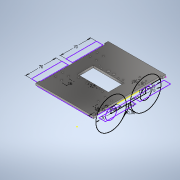
# Autodesk Inventor part: maze_02
Saved by Autodesk Inventor 2020 (Build 240168000, 168)
## iProperties
Created: 2022-07-14
Part Number: maze_02
Material: Сталь нержавеющая, 440C
Document SubType Name: Modeling
Designer: akapu
Density: 7.75 g/cm^3
Appearance: Сталь — полированная
Author: akapu
Autodesk Inventor part; units mm, degrees
ref_plane "YZ Plane" through (0, 0, 0) normal (1, 0, 0) x (0, 1, 0)
ref_plane "XZ Plane" through (0, 0, 0) normal (0, 1, 0) x (-1, 0, 0)
ref_plane "XY Plane" through (0, 0, 0) normal (0, 0, 1) x (1, 0, 0)
sketch "Эскиз2" plane through (0, 0, 0) normal (0, 1, 0) x (-1, 0, 0)
  line L0 (-37, -102) -> (-37, -192)
  line L1 (-166, -192) -> (-163, -192)
  line L2 (-163, -192) -> (-163, -102)
  line L3 (-37, -192) -> (-34, -192)
  line L4 (-34, -200) -> (-166, -200)
  line L5 (-37, -98) -> (-37, -102)
  line L6 (-163, -98) -> (-163, -102)
  line L7 (-166, -192) -> (-166, -200)
  line L8 (-34, -192) -> (-34, -200)
  line L9 (-163, -192) -> (-163, -157)
  line L10 (-163, -157) -> (-37, -157)
  line L11 (-163, -157) -> (-163, -63)
  line L12 (-163, -63) -> (-37, -63)
  line L13 (-34, -34.5) -> (-166, -34.5)
  line L14 (-166, -34.5) -> (-163, -34.5)
  line L15 (-163, -42.5) -> (-166, -42.5)
  line L16 (-166, -42.5) -> (-166, -34.5)
  line L17 (-34, -34.5) -> (-37, -34.5)
  line L18 (-37, -42.5) -> (-34, -42.5)
  line L19 (-37, -98) -> (-37, -34.5)
  line L20 (-34, -34.5) -> (-34, -42.5)
  line L21 (-163, -63) -> (-163, -34.5)
  point P0 (-37, -63)
  dimension "d181" = 94
  dimension "d247" = 8
  constraints: 44 end point, 5 parallel, 4 point on line, 3 horizontal, 3 perpendicular, 3 vertical
  measures "d181" distance of L9.end L11.end
  measures "d247" distance of L14.end L15.start
extrude "Выдавливание1" add sketch "Эскиз2" along normal blind 5
sketch "Эскиз3" plane through (0, 5, 0) normal (0, 1, 0) x (1, 0, 0)
  line L0 (163, 42.5) -> (163, 34.5)
  line L1 (34, 34.5) -> (166, 34.5) projected
  line L2 (156, 77.5) -> (156, 69.5)
  line L3 (166, 200) -> (34, 200) projected
  line L4 (156, 157) -> (156, 149)
  line L5 (156, 149) -> (142, 149)
  line L6 (142, 149) -> (142, 165)
  line L7 (142, 165) -> (156, 165)
  line L8 (156, 165) -> (156, 149)
  line L9 (156, 69.5) -> (142, 69.5)
  line L10 (142, 69.5) -> (142, 85.5)
  line L11 (142, 85.5) -> (156, 85.5)
  line L12 (156, 85.5) -> (156, 69.5)
  line L13 (37, 192) -> (37, 42.5) projected
  line L14 (44, 165) -> (58, 165)
  line L15 (58, 165) -> (58, 149)
  line L16 (58, 149) -> (44, 149)
  line L17 (44, 149) -> (44, 165)
  line L18 (58, 85.5) -> (44, 85.5)
  line L19 (44, 85.5) -> (44, 69.5)
  line L20 (44, 69.5) -> (58, 69.5)
  line L21 (58, 69.5) -> (58, 85.5)
  circle A0 centre (156, 69.5) radius 1.6
  circle A1 centre (142, 69.5) radius 1.6
  circle A2 centre (142, 85.5) radius 1.6
  circle A3 centre (156, 85.5) radius 1.6
  circle A4 centre (58, 69.5) radius 1.6
  circle A5 centre (58, 85.5) radius 1.6
  circle A6 centre (44, 69.5) radius 1.6
  circle A7 centre (44, 85.5) radius 1.6
  circle A8 centre (58, 149) radius 1.6
  circle A9 centre (58, 165) radius 1.6
  circle A10 centre (44, 149) radius 1.6
  circle A11 centre (44, 165) radius 1.6
  circle A12 centre (142, 165) radius 1.6
  circle A13 centre (142, 149) radius 1.6
  circle A14 centre (156, 149) radius 1.6
  circle A15 centre (156, 165) radius 1.6
  point P0 (0, 0)
  point P1 (37, 63)
  dimension "d255" = 14
  dimension "d256" = 16
  dimension "d260" = 14
  dimension "d261" = 3.2
  dimension "d262" = 3.2
  dimension "d263" = 3.2
  dimension "d264" = 3.2
  dimension "d265" = 3.2
  dimension "d266" = 3.2
  dimension "d267" = 3.2
  dimension "d268" = 3.2
  dimension "d269" = 3.2
  dimension "d270" = 3.2
  dimension "d271" = 3.2
  dimension "d272" = 3.2
  dimension "d273" = 3.2
  dimension "d274" = 3.2
  dimension "d275" = 3.2
  dimension "d276" = 3.2
  constraints: 38 end point, 16 centre point, 16 coincident, 8 parallel, 4 horizontal, 4 perpendicular, 3 point on line, 1 vertical
  measures "d255" distance of L6.end L7.end
  measures "d256" distance of L5.end L6.end
  measures "d260" distance of L15.end L16.end
  measures "d261" diameter of A0
  measures "d262" diameter of A1
  measures "d263" diameter of A2
  measures "d264" diameter of A3
  measures "d265" diameter of A4
  measures "d266" diameter of A5
  measures "d267" diameter of A6
  measures "d268" diameter of A7
  measures "d269" diameter of A8
  measures "d270" diameter of A9
  measures "d271" diameter of A10
  measures "d272" diameter of A11
  measures "d273" diameter of A12
  measures "d274" diameter of A13
  measures "d275" diameter of A14
  measures "d276" diameter of A15
extrude "Выдавливание2" cut sketch "Эскиз3" against normal blind 5 contours A0 L9 L2 | L2 L9 A0 | A3 L11 L12 | L12 L11 A3 | A1 L10 L9 | L9 L10 A1 | A2 L10 L11 | L11 L10 A2 | A14 L5 L4 | L4 L5 A14 | A15 L7 L8 | L8 L7 A15 | A13 L6 L5 | L5 L6 A13 | A12 L6 L7 | L7 L6 A12 | L17 A11 L14 | L14 A11 L17 | A9 L15 L14 | L14 L15 A9 | A10 L16 L17 | L17 L16 A10 | A8 L16 L15 | L15 L16 A8 | A7 L19 L18 | L18 L19 A7 | A5 L21 L18 | L18 L21 A5 | A6 L20 L19 | L19 L20 A6 | A4 L20 L21 | L21 L20 A4
sketch "Эскиз4" plane through (0, 0, 0) normal (0, -1, 0) x (1, 0, 0)
  line L0 (166, -200) -> (34, -200) projected
  line L1 (163, -157) -> (163, -170)
  line L2 (163, -170) -> (101.2, -170)
  line L3 (101.2, -170) -> (101.2, -144)
  line L4 (101.2, -144) -> (163, -144)
  line L5 (163, -144) -> (163, -170)
  line L6 (37, -170) -> (98.8, -170)
  line L7 (98.8, -170) -> (98.8, -144)
  line L8 (98.8, -144) -> (37, -144)
  line L9 (37, -144) -> (37, -170)
  line L10 (156, -157) -> (156, -165)
  line L11 (156, -165) -> (142, -165)
  line L12 (142, -165) -> (142, -149)
  line L13 (142, -149) -> (156, -149)
  line L14 (156, -149) -> (156, -165)
  line L15 (44, -165) -> (58, -165)
  line L16 (58, -165) -> (58, -149)
  line L17 (58, -149) -> (44, -149)
  line L18 (44, -149) -> (44, -165)
  line L19 (101.2, -144) -> (106.2, -144)
  line L20 (106.2, -90.5) -> (101.2, -90.5)
  line L21 (163, -41) -> (163, -192) projected
  line L22 (101.2, -90.5) -> (163, -90.5)
  line L23 (163, -90.5) -> (163, -64.5)
  line L24 (163, -64.5) -> (101.2, -64.5)
  line L25 (101.2, -64.5) -> (101.2, -90.5)
  line L26 (37, -192) -> (37, -42.5) projected
  line L27 (98.8, -90.5) -> (37, -90.5)
  line L28 (37, -90.5) -> (37, -64.5)
  line L29 (37, -64.5) -> (98.8, -64.5)
  line L30 (98.8, -64.5) -> (98.8, -90.5)
  line L31 (44, -77.5) -> (44, -85.5)
  circle A0 centre (58, -71) radius 1.6 projected
  line L32 (44, -85.5) -> (58.5568, -85.5)
  line L33 (58.5568, -85.5) -> (58.5568, -69.5)
  line L34 (58.5568, -69.5) -> (44, -69.5)
  line L35 (44, -69.5) -> (44, -85.5)
  circle A1 centre (142, -71) radius 1.6 projected
  line L36 (156, -85.5) -> (142, -85.5)
  line L37 (142, -85.5) -> (142, -69.4)
  line L38 (142, -69.4) -> (156, -69.4)
  line L39 (156, -69.4) -> (156, -85.5)
  line L40 (163, -77.5) -> (163, -34.5)
  line L41 (163, -34.5) -> (37, -34.5)
  line L42 (37, -34.5) -> (37, -41)
  line L43 (163, -157) -> (170, -157)
  line L44 (170, -157) -> (170, -192)
  line L45 (163, -77.5) -> (170, -77.5)
  line L46 (170, -77.5) -> (170, -42.5)
  line L47 (37, -77.5) -> (30, -77.5)
  line L48 (30, -77.5) -> (30, -42.5)
  line L49 (30, -42.5) -> (15, -42.5)
  line L50 (15, -42.5) -> (15, -112.5)
  line L51 (15, -112.5) -> (30, -112.5)
  line L52 (30, -112.5) -> (30, -42.5)
  line L53 (170, -42.5) -> (185, -42.5)
  line L54 (185, -42.5) -> (185, -112.5)
  line L55 (185, -112.5) -> (170, -112.5)
  line L56 (170, -112.5) -> (170, -42.5)
  line L57 (37, -157) -> (30, -157)
  line L58 (30, -192) -> (15, -192)
  line L59 (15, -192) -> (15, -122)
  line L60 (15, -122) -> (30, -122)
  line L61 (30, -122) -> (30, -192)
  line L62 (170, -192) -> (185, -192)
  line L63 (185, -192) -> (185, -122)
  line L64 (185, -122) -> (170, -122)
  line L65 (170, -122) -> (170, -192)
  point P0 (142, -155)
  point P1 (44, -155)
  point P2 (37, -63)
  dimension "d162" = 8
  dimension "d163" = 16
  dimension "d240" = 26
  dimension "d241" = 2.4
  dimension "d243" = 16
  dimension "d244" = 14
  dimension "d245" = 43
  dimension "d284" = 70
  dimension "d286" = 70
  constraints: 126 end point, 25 parallel, 17 perpendicular, 14 horizontal, 7 point on line, 2 midpoint, 1 vertical, 1 vertical alignment, 3 other
  measures "d162" distance of L10.start L10.end
  measures "d163" distance of L11.end L12.end
  measures "d240" distance of L23.end L22.end
  measures "d241" distance of L20.end L27.start
  measures "d243" distance of L33.end L32.end
  measures "d244" distance of L37.end L38.end
  measures "d245" distance of L40.start L40.end
  measures "d284" distance of L50.end L49.end
  measures "d286" distance of L58.end L59.end
sketch "Эскиз11" plane through (163, 0, -42.5) normal (1, 0, 0) x (0, 0, -1)
  line L0 (0, 0) -> (149.5, 0) projected
  line L1 (0, 0) -> (35, 0)
  line L2 (35, 0) -> (35, -12.5)
  line L3 (149.5, 0) -> (114.5, 0)
  line L4 (114.5, 0) -> (114.5, -12.5)
  line L5 (114.5, -12.5) -> (35, -12.5)
  circle A0 centre (35, -12.5) radius 35
  circle A1 centre (114.5, -12.5) radius 35
  line L6 (59.7487, -37.2487) -> (74.75, -22.2475)
  line L7 (74.75, -22.2475) -> (89.7513, -37.2487)
  line L8 (74.75, -22.2475) -> (74.75, -12.5)
  circle A2 centre (35, -12.5) radius 12.5
  circle A3 centre (114.5, -12.5) radius 12.5
  point P0 (-42.5, 0)
  dimension "d291" = 70
  dimension "d292" = 70
  dimension "d287" = 35
  dimension "d288" = 12.5
  dimension "d289" = 35
  dimension "d290" = 12.5
  dimension "d321" = 90
  dimension "d322" = 9.7475
  constraints: 16 end point, 3 coincident, 2 perpendicular, 2 point on line, 2 vertical alignment, 1 midpoint, 12 other
  measures "d287" distance of L0.start L1.end
  measures "d288" distance of L1.end L2.end
  measures "d289" distance of L0.end L3.end
  measures "d290" distance of L3.end L4.end
  measures "d321" angle of L7 L6
  measures "d322" distance of L6.end L8.end
sketch "Эскиз12" plane through (0, 0, 0) normal (0, -1, 0) x (1, 0, 0)
  line L0 (37, -192) -> (37, -42.5) projected
  line L1 (34, -34.5) -> (166, -34.5) projected
  line L2 (37, -34.5) -> (37, -77.5)
  line L3 (37, -77.5) -> (98.8, -77.5)
  line L4 (98.8, -77.5) -> (98.8, -90.5)
  line L5 (98.8, -90.5) -> (93.8, -90.5)
  line L6 (100, -99.25) -> (64.5, -99.25)
  line L7 (64.5, -99.25) -> (135.5, -99.25)
  line L8 (135.5, -99.25) -> (135.5, -135.25)
  line L9 (135.5, -135.25) -> (64.5, -135.25)
  line L10 (64.5, -135.25) -> (64.5, -99.25)
  line L11 (106.2, -141) -> (93.8, -141)
  circle A0 centre (106.2, -141) radius 3
  circle A1 centre (93.8, -141) radius 3
  line L12 (106.2, -93.5) -> (93.8, -93.5)
  circle A2 centre (106.2, -93.5) radius 3
  circle A3 centre (93.8, -93.5) radius 3
  point P0 (0, 0)
  dimension "d296" = 43
  dimension "d298" = 13
  dimension "d310" = 35.5
  dimension "d311" = 71
  dimension "d312" = 36
  dimension "d343" = 6
  dimension "d344" = 6
  dimension "d346" = 6
  dimension "d347" = 6
  constraints: 22 end point, 4 centre point, 4 coincident, 4 perpendicular, 2 parallel, 2 point on line, 1 horizontal
  measures "d296" distance of L2.start L2.end
  measures "d298" distance of L3.end L4.end
  measures "d310" distance of L6.start L6.end
  measures "d311" distance of L8.end L9.end
  measures "d312" distance of L7.end L8.end
  measures "d343" diameter of A0
  measures "d344" diameter of A1
  measures "d346" diameter of A2
  measures "d347" diameter of A3
extrude "Выдавливание9" cut sketch "Эскиз12" against normal blind 5
sketch "Эскиз13" plane through (0, 0, 0) normal (0, -1, 0) x (1, 0, 0)
  line L0 (135.5, -135.25) -> (135.5, -99.25) projected
  line L1 (135.5, -99.25) -> (135.5, -90.5)
  line L2 (135.5, -135.25) -> (64.5, -135.25) projected
  line L3 (64.5, -135.25) -> (64.5, -144)
  line L4 (64.5, -144) -> (135.5, -144)
  line L5 (135.5, -144) -> (135.5, -90.5)
  line L6 (135.5, -90.5) -> (64.5, -90.5)
  line L7 (64.5, -90.5) -> (64.5, -144)
  line L8 (135.5, -90.5) -> (127.5, -90.5)
  line L9 (127.5, -90.5) -> (127.5, -93.5)
  line L10 (127.5, -93.5) -> (135.5, -93.5)
  line L11 (135.5, -93.5) -> (135.5, -90.5)
  line L12 (64.5, -144) -> (72.5, -144)
  line L13 (72.5, -144) -> (72.5, -141)
  line L14 (72.5, -141) -> (64.5, -141)
  line L15 (64.5, -141) -> (64.5, -144)
  line L16 (72.5, -141) -> (127.5, -141)
  line L17 (127.5, -141) -> (127.5, -93.5)
  line L18 (127.5, -93.5) -> (72.5, -93.5)
  line L19 (72.5, -93.5) -> (72.5, -141)
  circle A0 centre (127.5, -93.5) radius 1.6
  circle A1 centre (127.5, -141) radius 1.6
  circle A2 centre (72.5, -141) radius 1.6
  circle A3 centre (72.5, -93.5) radius 1.6
  point P0 (163, -42.5)
  dimension "d325" = 8.75
  dimension "d326" = 8.75
  dimension "d327" = 8
  dimension "d328" = 3
  dimension "d329" = 8
  dimension "d330" = 3
  dimension "d331" = 3.2
  dimension "d332" = 3.2
  dimension "d333" = 3.2
  dimension "d334" = 3.2
  constraints: 36 end point, 8 parallel, 4 centre point, 4 coincident, 4 horizontal, 4 perpendicular, 2 vertical
  measures "d325" distance of L0.end L1.end
  measures "d326" distance of L2.end L3.end
  measures "d327" distance of L10.end L9.end
  measures "d328" distance of L9.end L8.end
  measures "d329" distance of L14.end L13.end
  measures "d330" distance of L13.end L12.end
  measures "d331" diameter of A0
  measures "d332" diameter of A1
  measures "d333" diameter of A2
  measures "d334" diameter of A3
extrude "Выдавливание10" cut sketch "Эскиз13" against normal blind 5 contours A1 L16 L17 | L17 L16 A1 | A0 L18 L17 | L17 L10 A0 | L10 L9 A0 | A3 L18 L19 | L19 L18 A3 | A2 L16 L19 | L19 L14 A2 | L18 A0 L9 | A2 L14 L13 | L13 L16 A2
sketch "Эскиз15" plane through (0, 5, 0) normal (0, 1, 0) x (1, 0, 0)
  line L0 (72.5, 93.5) -> (80.5, 93.5)
  line L1 (80.5, 93.5) -> (80.5, 96.3)
  line L2 (80.5, 96.3) -> (72.5, 96.3)
  line L3 (72.5, 96.3) -> (72.5, 93.5)
  circle A0 centre (127.5, 93.5) radius 1.6 projected
  line L4 (127.5, 93.5) -> (119.5, 93.5)
  line L5 (119.5, 93.5) -> (119.5, 96.3)
  line L6 (119.5, 96.3) -> (127.5, 96.3)
  line L7 (127.5, 96.3) -> (127.5, 93.5)
  circle A1 centre (127.5, 141) radius 1.6 projected
  line L8 (127.5, 141) -> (119.5, 141)
  line L9 (119.5, 141) -> (119.5, 138.2)
  line L10 (119.5, 138.2) -> (127.5, 138.2)
  line L11 (127.5, 138.2) -> (127.5, 141)
  line L12 (72.5, 141) -> (80.5, 141)
  line L13 (80.5, 141) -> (80.5, 138.2)
  line L14 (80.5, 138.2) -> (72.5, 138.2)
  line L15 (72.5, 138.2) -> (72.5, 141)
  circle A2 centre (80.5, 138.2) radius 1.6
  circle A3 centre (119.5, 138.2) radius 1.6
  circle A4 centre (119.5, 96.3) radius 1.6
  circle A5 centre (80.5, 96.3) radius 1.6
  point P0 (0, 0)
  dimension "d348" = 8
  dimension "d349" = 2.8
  dimension "d350" = 8
  dimension "d351" = 2.8
  dimension "d352" = 8
  dimension "d353" = 2.8
  dimension "d354" = 3.2
  dimension "d355" = 3.2
  dimension "d356" = 3.2
  dimension "d357" = 3.2
  constraints: 32 end point, 8 parallel, 4 centre point, 4 coincident, 4 horizontal, 4 perpendicular, 4 point on line
  measures "d348" distance of L2.end L1.end
  measures "d349" distance of L1.end L0.end
  measures "d350" distance of L5.end L6.end
  measures "d351" distance of L4.end L5.end
  measures "d352" distance of L10.end L9.end
  measures "d353" distance of L9.end L8.end
  measures "d354" diameter of A2
  measures "d355" diameter of A3
  measures "d356" diameter of A4
  measures "d357" diameter of A5
extrude "Выдавливание12" cut sketch "Эскиз15" against normal blind 5 contours A5 L2 L1 | L1 L2 A5 | A4 L5 L6 | L6 L5 A4 | A3 L10 L9 | L9 L10 A3 | A2 L14 L13 | L13 L14 A2
fillet "Сопряжение3" radius 1.2 4 edges at (78.9, 0, -96.3) (117.9, 0, -96.3) (117.9, 0, -138.2) (78.9, 0, -138.2) inverted yes
